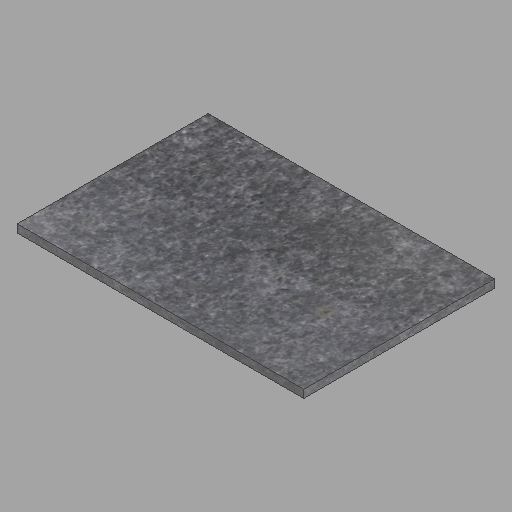
# Autodesk Inventor part: 1xRNDxRND-1074sqft
Saved by Autodesk Inventor 2023 (Build 270158000, 158)
## iProperties
Created: 2022-02-10
Part Number: 1xRNDxRND-1074sqft
Material: Granite, Cut, Polished
Document SubType Name: Modeling
Designer: awelt
Density: 2.7 g/cm^3
Appearance: Kasota SN sapphire
Mass: 38227.7 g
Surface Area: 11922.6 cm^2
Volume: 14158.4 cm^3
TEST: 0.0
Author: awelt
Autodesk Inventor part; units mm, degrees
ref_plane "YZ Plane" through (0, 0, 0) normal (1, 0, 0) x (0, 1, 0)
ref_plane "XZ Plane" through (0, 0, 0) normal (0, 1, 0) x (-1, 0, 0)
ref_plane "XY Plane" through (0, 0, 0) normal (0, 0, 1) x (1, 0, 0)
sketch "Sketch3" plane through (0, 0, 0) normal (0, 1, 0) x (-1, 0, 0)
  line L0 (457.2, -304.8) -> (-457.2, -304.8)
  line L1 (-457.2, -304.8) -> (-457.2, 304.8)
  line L2 (-457.2, 304.8) -> (457.2, 304.8)
  line L3 (457.2, 304.8) -> (457.2, -304.8)
  line L4 (457.2, -304.8) -> (-457.2, 304.8) construction
  line L5 (-457.2, -304.8) -> (457.2, 304.8) construction
  point P0 (0, 0)
  dimension "d4" = 914.4
  dimension "d5" = 609.6
  constraints: 12 end point, 2 midpoint, 2 parallel, 1 horizontal, 1 perpendicular
  measures "d4" distance of L1.end L2.end
  measures "d5" distance of L0.end L1.end
extrude "Extrusion2" add sketch "Sketch3" along normal blind 25.4
body "Solid2"
